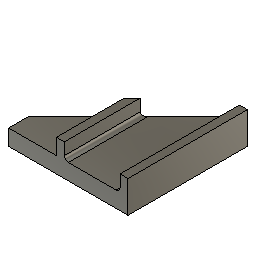
Frame Squaring Tool Parametric (Autodesk Fusion 360 design; units mm, degrees)
Autodesk Fusion 360 part; units mm, degrees
sketch "Sketch5" plane through (0, 0, 0) normal (0, 1, 0) x (1, 0, 0)
  line L0 (150, 0) -> (150, -40)
  line L1 (150, -40) -> (140, -40)
  line L2 (140, -40) -> (140, -25)
  line L3 (150, 0) -> (150, -40)
  line L4 (70.1, -40) -> (70.1, -25)
  line L5 (75.1, -20) -> (135, -20)
  line L6 (140, -25) -> (140, -40)
  line L7 (70.1, -40) -> (60.1, -40)
  line L8 (60.1, -40) -> (60.1, -20)
  line L9 (70.1, -25) -> (70.1, -40)
  line L10 (150, -40) -> (140, -40)
  line L11 (70.1, -40) -> (60.1, -40)
  arc A0 (75.1, -20) -> (70.1, -25) centre (75.1, -25) ccw
  arc A1 (140, -25) -> (135, -20) centre (135, -25) ccw
  line L12 (0, 0) -> (0, -20)
  line L13 (0, -20) -> (60.1, -20)
  line L14 (0, 0) -> (150, 0)
  dimension "d18" = 10
  dimension "d19" = 69.9
  dimension "d20" = 10
  dimension "d21" = 5
  dimension "d24" = 150
  dimension "d34" = 40
  dimension "d35" = 20
  constraint vertical L0
  constraint horizontal L10
  constraint horizontal L1
  constraint vertical L2
  constraint vertical L3
  constraint vertical L4
  constraint horizontal L5
  constraint vertical L6
  constraint horizontal L7
  constraint vertical L8
  constraint vertical L9
  constraint collinear L10 L11
  constraint tangent L5 A0
  constraint tangent L4 A0
  constraint tangent L6 A1
  constraint tangent L5 A1
  constraint equal A0 A1
  constraint vertical L12
  constraint horizontal L13
  constraint perpendicular L0 L14
  measures "d18" distance of L0.end L1.end
  measures "d19" distance of L1.end L4.start
  measures "d20" distance of L4.start L7.end
  measures "d21" radius of A0
  measures "d24" distance of L0.start L12.start
  measures "d34" distance of L0.start L0.end
  measures "d35" distance of L12.start L12.end
extrude "Extrude5" add sketch "Sketch5" along normal blind 150
sketch "Sketch6" plane through (0, 0, 0) normal (0, 0, -1) x (1, 0, 0)
  line L0 (150, 0) -> (0, 0)
  line L1 (0, 0) -> (0, -150)
  line L2 (0, -150) -> (150, -150)
  line L3 (150, -150) -> (150, 0)
  line L4 (0, -150) -> (125, -150)
  line L5 (125, -150) -> (125, -25)
  line L6 (125, -25) -> (0, -25)
  line L7 (0, -25) -> (0, -150)
  line L8 (0, -25) -> (125, -150)
  dimension "d29" = 125
  dimension "d30" = 125
  constraint horizontal L4
  constraint vertical L5
  constraint horizontal L6
  constraint vertical L7
  constraint coincident L1.end L2.start
  measures "d29" distance of L1.end L4.end
  measures "d30" distance of L1.end L6.end
extrude "Extrude6" cut sketch "Sketch6" against normal up to surface (40 mm away) contours L1 L2 L4 L7 L8
equation "ExtrusionRadius = 5 mm"
equation "ExtrusionWidth = 69.9 mm"
equation "d18 = WallWidth"
equation "d19 = ExtrusionWidth"
equation "d20 = WallWidth"
equation "d21 = ExtrusionRadius"
equation "WallWidth = 10 mm"
equation "d24 = Base"
equation "Base = 150 mm"
equation "d26 = Base"
equation "BaseCorner = Base - 25 mm"
equation "d29 = BaseCorner"
equation "d30 = BaseCorner"
equation "ToolHeight = 40 mm"
equation "d34 = ToolHeight"
equation "d35 = ToolHeight / 2"
named bodies: "Frame Squaring Tool"
